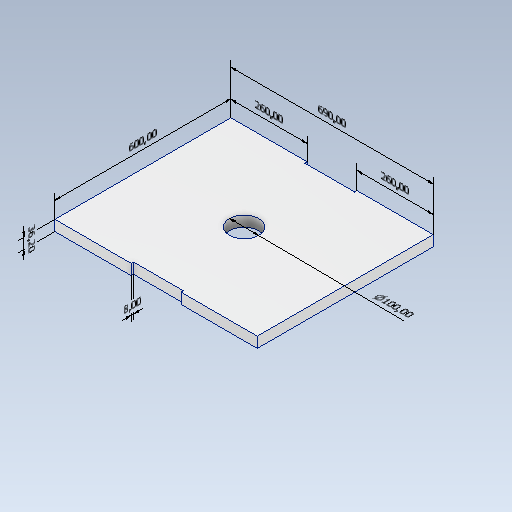
# Autodesk Inventor part: piso
Saved by Autodesk Inventor 2021 (Build 250183000, 183)
## iProperties
Created: 2020-10-29
Part Number: piso
Material: Aluminio 6061
Document SubType Name: Modeling
Designer: germi
Density: 2.7 g/cm^3
Appearance: Aluminio - Plano
Mass: 39430.9 g
Surface Area: 9127.79 cm^2
Volume: 14604 cm^3
Author: germi
Autodesk Inventor part; units mm, degrees
ref_plane "YZ Plane" through (0, 0, 0) normal (1, 0, 0) x (0, 1, 0)
ref_plane "XZ Plane" through (0, 0, 0) normal (0, 1, 0) x (-1, 0, 0)
ref_plane "XY Plane" through (0, 0, 0) normal (0, 0, 1) x (1, 0, 0)
sketch "Boceto1" plane through (0, 0, 0) normal (0, 1, 0) x (-1, 0, 0)
  line L0 (-690, 0) -> (-690, -628.4316)
  line L1 (0, -628.4316) -> (0, 0)
  line L2 (-430, 0) -> (-430, -8)
  line L3 (-430, -8) -> (-260, -8)
  line L4 (-260, -8) -> (-260, 0)
  line L5 (-260, -592) -> (-430, -592)
  line L6 (0, 0) -> (-260, 0)
  line L7 (-430, 0) -> (-690, 0)
  line L8 (-690, -600) -> (-430, -600)
  line L9 (-260, -600) -> (0, -600)
  line L10 (-430, -592) -> (-430, -600)
  line L11 (-260, -592) -> (-260, -600)
  point P0 (0, -600)
  point P1 (-345, -300)
  dimension "d32" = 600
  dimension "d33" = 690
  constraints: 24 end point, 6 parallel, 3 perpendicular, 2 horizontal, 1 vertical
  measures "d32" distance between parallel lines of L6 L9
  measures "d33" distance between parallel lines of L0 L1
extrude "Extrusión1" add sketch "Boceto1" along normal blind 36.2
sketch "Boceto2" plane through (0, 36.2, 0) normal (0, 1, 0) x (1, 0, 0)
  line L0 (260, 600) -> (0, 600) projected
  line L1 (0, 600) -> (0, 0) projected
  point P0 (345, 300)
hole "Agujero1" at (345, 36.2, -300) direction (0, -1, 0) diameter 100 end through all
